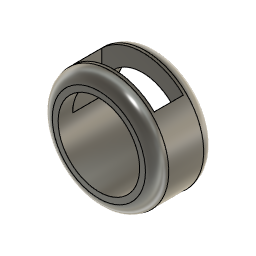
Collimating Ring (Autodesk Fusion 360 design; units mm, degrees)
Autodesk Fusion 360 part; units mm, degrees
sketch "Sketch1" plane through (0, 0, 0) normal (0, 1, 0) x (1, 0, 0)
  circle A0 centre (0, 0) radius 3.5
  circle A1 centre (0, 0) radius 5
  dimension "d1" = 7
  dimension "d2" = 10
  constraint coincident A0.centre A1.centre
  constraint concentric A0 A1
  measures "d1" diameter of A0
  measures "d2" diameter of A1
extrude "Extrude1" add sketch "Sketch1" along normal blind 3 and the other way blind 2
sketch "Sketch2" plane through (0, 0, 0) normal (0, 0, 1) x (1, 0, 0)
  line L0 (3.5, -0.75) -> (-3.5, -0.75)
  line L1 (-3.5, -0.75) -> (-3.5, 1.75)
  line L2 (-3.5, 1.75) -> (3.5, 1.75)
  line L3 (3.5, 1.75) -> (3.5, -0.75)
  line L4 (0, 0) -> (-3.5, 0)
  line L5 (0, 0) -> (0, 1.75)
  dimension "d7" = 7
  dimension "d8" = 2.5
  dimension "d15" = 3.5
  dimension "d16" = 1.75
  constraint horizontal L0
  constraint vertical L1
  constraint horizontal L2
  constraint vertical L3
  constraint coincident L4.start L5.start
  constraint coincident L1 L4.end
  constraint perpendicular L1 L4
  constraint coincident L2 L5.end
  constraint perpendicular L2 L5
  measures "d7" distance of L0.start L0.end
  measures "d8" distance of L0.start L2.end
  measures "d15" distance of L4.start L4.end
  measures "d16" distance of L4.start L5.end
extrude "Extrude2" cut sketch "Sketch2" along normal blind 5
fillet "Fillet1" radius 1 1 edges at (-4.6616, 3, 1.8081)
fillet "Fillet2" radius 1 1 edges at (-4.6616, -2, -1.8081)
